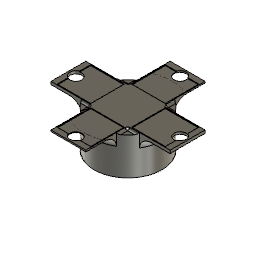
SpincoatG3P-8_rotor_4x_22x22coverslips_v1 (Autodesk Fusion 360 design; units mm, degrees)
Autodesk Fusion 360 part; units mm, degrees
sketch "Sketch1" plane through (0, 0, 0) normal (0, 0, 1) x (1, 0, 0)
  circle A0 centre (0, 0) radius 22.75
  dimension "d1" = 45.5
  constraint coincident A0.centre origin
  measures "d1" diameter of A0
extrude "Extrude1" add sketch "Sketch1" along normal blind 25
sketch "Sketch2" plane through (0, 0, 0) normal (0, 0, -1) x (1, 0, 0)
  circle A0 centre (0, 0) radius 22.75
  circle A1 centre (0, 0) radius 22.25
  dimension "d4" = 44.5
  constraint concentric A0 A1
  measures "d4" diameter of A1
extrude "Extrude2" cut sketch "Sketch2" against normal blind 10 contours A1
sketch "Sketch3" plane through (0, 0, 25) normal (0, 0, 1) x (-1, 0, 0)
  circle A0 centre (0, 0) radius 22.75
  line L0 (11.75, -27.5) -> (-11.75, -27.5)
  line L1 (-11.75, -27.5) -> (-11.75, 27.5)
  line L2 (-11.75, 27.5) -> (11.75, 27.5)
  line L3 (11.75, 27.5) -> (11.75, -27.5)
  line L4 (11.75, -27.5) -> (-11.75, 27.5) construction
  line L5 (-11.75, -27.5) -> (11.75, 27.5) construction
  dimension "d7" = 23.5
  dimension "d8" = 55
  constraint horizontal L0
  constraint perpendicular L0 L1
  constraint parallel L0 L2
  constraint parallel L1 L3
  constraint coincident L4 A0.centre
  constraint coincident L5 A0.centre
  constraint coincident A0.centre origin
  measures "d7" distance of L1.end L2.end
  measures "d8" distance of L0.end L1.end
sketch "Sketch6" plane through (0, 0, 25) normal (0, 0, 1) x (-1, 0, 0)
  circle A0 centre (0, 0) radius 22.75
  line L0 (-11.75, 40) -> (11.75, 40)
  line L1 (11.75, 40) -> (11.75, -40)
  line L2 (11.75, -40) -> (-11.75, -40)
  line L3 (-11.75, -40) -> (-11.75, 40)
  line L4 (-11.75, 40) -> (11.75, -40) construction
  line L5 (11.75, 40) -> (-11.75, -40) construction
  dimension "d17" = 23.5
  dimension "d18" = 80
  constraint horizontal L0
  constraint perpendicular L0 L1
  constraint parallel L0 L2
  constraint parallel L1 L3
  constraint coincident L4 A0.centre
  constraint coincident L5 A0.centre
  constraint coincident A0.centre origin
  measures "d17" distance of L1.end L2.end
  measures "d18" distance of L0.end L1.end
extrude "Extrude6" add sketch "Sketch6" along normal blind 1 contours A0 L1 L3 | A0 L0 L1 L3 | A0 L1 L2 L3
sketch "Sketch7" plane through (0, 0, 26) normal (0, 0, 1) x (-1, 0, 0)
  line L0 (-11.75, -40) -> (11.75, -40)
  line L1 (11.75, -40) -> (11.75, 40)
  line L2 (11.75, 40) -> (-11.75, 40)
  line L3 (-11.75, 40) -> (-11.75, -40)
  line L4 (-40, 11.75) -> (40, 11.75)
  line L5 (40, 11.75) -> (40, -11.75)
  line L6 (40, -11.75) -> (-40, -11.75)
  line L7 (-40, -11.75) -> (-40, 11.75)
  line L8 (-40, 11.75) -> (40, -11.75) construction
  line L9 (40, 11.75) -> (-40, -11.75) construction
  dimension "d21" = 80
  dimension "d22" = 23.5
  constraint horizontal L4
  constraint perpendicular L4 L5
  constraint parallel L4 L6
  constraint parallel L5 L7
  constraint coincident L8 origin
  constraint coincident L9 origin
  measures "d21" distance of L5.end L6.end
  measures "d22" distance of L4.end L5.end
extrude "Extrude7" add sketch "Sketch7" against normal blind 2 contours L3 L4 L6 L7 | L1 L3 L4 L6 | L1 L4 L5 L6
sketch "Sketch8" plane through (0, 0, 26) normal (0, 0, 1) x (-1, 0, 0)
  line L0 (11.75, 11.75) -> (11.75, 40)
  line L1 (11.75, 40) -> (-11.75, 40)
  line L2 (-11.75, 40) -> (-11.75, 11.75)
  line L3 (-11.75, 11.75) -> (-40, 11.75)
  line L4 (-40, 11.75) -> (-40, -11.75)
  line L5 (-40, -11.75) -> (-11.75, -11.75)
  line L6 (-11.75, -11.75) -> (-11.75, -40)
  line L7 (-11.75, -40) -> (11.75, -40)
  line L8 (11.75, -40) -> (11.75, -11.75)
  line L9 (11.75, -11.75) -> (40, -11.75)
  line L10 (40, -11.75) -> (40, 11.75)
  line L11 (40, 11.75) -> (11.75, 11.75)
  line L12 (-11.25, 36.25) -> (11.25, 36.25)
  line L13 (11.25, 36.25) -> (11.25, 13.75)
  line L14 (11.25, 13.75) -> (-11.25, 13.75)
  line L15 (-11.25, 13.75) -> (-11.25, 36.25)
  line L16 (-11.25, 36.25) -> (11.25, 13.75) construction
  line L17 (11.25, 36.25) -> (-11.25, 13.75) construction
  point P0 (0, 25)
  dimension "d25" = 22.5
  dimension "d26" = 22.5
  constraint horizontal L12
  constraint perpendicular L12 L13
  constraint parallel L12 L14
  constraint parallel L13 L15
  constraint coincident L16 P0
  constraint coincident L17 P0
  measures "d25" distance of L13.end L14.end
  measures "d26" distance of L12.end L13.end
extrude "Extrude8" cut sketch "Sketch8" against normal blind 0.5 contours L12 L13 L14 L15
sketch "Sketch9" plane through (0, 0, 26) normal (0, 0, 1) x (-1, 0, 0)
  line L0 (11.25, 36.25) -> (11.25, 13.75)
  line L1 (11.25, 13.75) -> (-11.25, 13.75)
  line L2 (-11.25, 13.75) -> (-11.25, 36.25)
  line L3 (-11.25, 36.25) -> (11.25, 36.25)
  line L4 (11.75, 11.75) -> (11.75, 40)
  line L5 (11.75, 40) -> (-11.75, 40)
  line L6 (-11.75, 40) -> (-11.75, 11.75)
  line L7 (-11.75, 11.75) -> (-40, 11.75)
  line L8 (-40, 11.75) -> (-40, -11.75)
  line L9 (-40, -11.75) -> (-11.75, -11.75)
  line L10 (-11.75, -11.75) -> (-11.75, -40)
  line L11 (-11.75, -40) -> (11.75, -40)
  line L12 (11.75, -40) -> (11.75, -11.75)
  line L13 (11.75, -11.75) -> (40, -11.75)
  line L14 (40, -11.75) -> (40, 11.75)
  line L15 (40, 11.75) -> (11.75, 11.75)
  line L16 (36.25, -11.25) -> (13.75, -11.25)
  line L17 (13.75, -11.25) -> (13.75, 11.25)
  line L18 (13.75, 11.25) -> (36.25, 11.25)
  line L19 (36.25, 11.25) -> (36.25, -11.25)
  line L20 (36.25, -11.25) -> (13.75, 11.25) construction
  line L21 (13.75, -11.25) -> (36.25, 11.25) construction
  point P0 (25, 0)
  dimension "d29" = 22.5
  dimension "d30" = 22.5
  constraint horizontal L16
  constraint perpendicular L16 L17
  constraint parallel L16 L18
  constraint parallel L17 L19
  constraint coincident L20 P0
  constraint coincident L21 P0
  measures "d29" distance of L17.end L18.end
  measures "d30" distance of L16.end L17.end
extrude "Extrude9" cut sketch "Sketch9" against normal blind 0.5 contours L16 L17 L18 L19
sketch "Sketch10" plane through (0, 0, 26) normal (0, 0, 1) x (-1, 0, 0)
  line L0 (13.75, -11.25) -> (13.75, 11.25)
  line L1 (13.75, 11.25) -> (36.25, 11.25)
  line L2 (36.25, 11.25) -> (36.25, -11.25)
  line L3 (36.25, -11.25) -> (13.75, -11.25)
  line L4 (11.25, 36.25) -> (11.25, 13.75)
  line L5 (11.25, 13.75) -> (-11.25, 13.75)
  line L6 (-11.25, 13.75) -> (-11.25, 36.25)
  line L7 (-11.25, 36.25) -> (11.25, 36.25)
  line L8 (11.75, 11.75) -> (11.75, 40)
  line L9 (11.75, 40) -> (-11.75, 40)
  line L10 (-11.75, 40) -> (-11.75, 11.75)
  line L11 (-11.75, 11.75) -> (-40, 11.75)
  line L12 (-40, 11.75) -> (-40, -11.75)
  line L13 (-40, -11.75) -> (-11.75, -11.75)
  line L14 (-11.75, -11.75) -> (-11.75, -40)
  line L15 (-11.75, -40) -> (11.75, -40)
  line L16 (11.75, -40) -> (11.75, -11.75)
  line L17 (11.75, -11.75) -> (40, -11.75)
  line L18 (40, -11.75) -> (40, 11.75)
  line L19 (40, 11.75) -> (11.75, 11.75)
  line L20 (-11.25, -36.25) -> (11.25, -36.25)
  line L21 (11.25, -36.25) -> (11.25, -13.75)
  line L22 (11.25, -13.75) -> (-11.25, -13.75)
  line L23 (-11.25, -13.75) -> (-11.25, -36.25)
  line L24 (-11.25, -36.25) -> (11.25, -13.75) construction
  line L25 (11.25, -36.25) -> (-11.25, -13.75) construction
  point P0 (0, -25)
  dimension "d33" = 22.5
  dimension "d34" = 22.5
  constraint horizontal L20
  constraint perpendicular L20 L21
  constraint parallel L20 L22
  constraint parallel L21 L23
  constraint coincident L24 P0
  constraint coincident L25 P0
  measures "d33" distance of L21.end L22.end
  measures "d34" distance of L20.end L21.end
extrude "Extrude10" cut sketch "Sketch10" against normal blind 0.5 contours L20 L21 L22 L23
sketch "Sketch11" plane through (0, 0, 26) normal (0, 0, 1) x (-1, 0, 0)
  line L0 (11.25, -36.25) -> (-11.25, -36.25)
  line L1 (-11.25, -36.25) -> (-11.25, -13.75)
  line L2 (-11.25, -13.75) -> (11.25, -13.75)
  line L3 (11.25, -13.75) -> (11.25, -36.25)
  line L4 (13.75, -11.25) -> (13.75, 11.25)
  line L5 (13.75, 11.25) -> (36.25, 11.25)
  line L6 (36.25, 11.25) -> (36.25, -11.25)
  line L7 (36.25, -11.25) -> (13.75, -11.25)
  line L8 (11.25, 36.25) -> (11.25, 13.75)
  line L9 (11.25, 13.75) -> (-11.25, 13.75)
  line L10 (-11.25, 13.75) -> (-11.25, 36.25)
  line L11 (-11.25, 36.25) -> (11.25, 36.25)
  line L12 (11.75, 11.75) -> (11.75, 40)
  line L13 (11.75, 40) -> (-11.75, 40)
  line L14 (-11.75, 40) -> (-11.75, 11.75)
  line L15 (-11.75, 11.75) -> (-40, 11.75)
  line L16 (-40, 11.75) -> (-40, -11.75)
  line L17 (-40, -11.75) -> (-11.75, -11.75)
  line L18 (-11.75, -11.75) -> (-11.75, -40)
  line L19 (-11.75, -40) -> (11.75, -40)
  line L20 (11.75, -40) -> (11.75, -11.75)
  line L21 (11.75, -11.75) -> (40, -11.75)
  line L22 (40, -11.75) -> (40, 11.75)
  line L23 (40, 11.75) -> (11.75, 11.75)
  line L24 (-36.25, 11.25) -> (-13.75, 11.25)
  line L25 (-13.75, 11.25) -> (-13.75, -11.25)
  line L26 (-13.75, -11.25) -> (-36.25, -11.25)
  line L27 (-36.25, -11.25) -> (-36.25, 11.25)
  line L28 (-36.25, 11.25) -> (-13.75, -11.25) construction
  line L29 (-13.75, 11.25) -> (-36.25, -11.25) construction
  point P0 (-25, 0)
  dimension "d37" = 22.5
  dimension "d38" = 22.5
  constraint horizontal L24
  constraint perpendicular L24 L25
  constraint parallel L24 L26
  constraint parallel L25 L27
  constraint coincident L28 P0
  constraint coincident L29 P0
  measures "d37" distance of L25.end L26.end
  measures "d38" distance of L24.end L25.end
extrude "Extrude11" cut sketch "Sketch11" against normal blind 0.5 contours L24 L25 L26 L27
sketch "Sketch12" plane through (0, 0, 24) normal (0, 0, -1) x (1, 0, 0)
  arc A0 (-19.4808, 11.75) -> (-19.4808, -11.75) centre (0, 0) ccw
  line L0 (-19.4808, 11.75) -> (-40, 11.75)
  line L1 (-40, 11.75) -> (-40, -11.75)
  line L2 (-40, -11.75) -> (-19.4808, -11.75)
  circle A1 centre (-35, 0) radius 4
  dimension "d41" = 8
  measures "d41" diameter of A1
extrude "Extrude12" cut sketch "Sketch12" against normal blind 10 contours A1
sketch "Sketch13" plane through (0, 0, 25) normal (0, 0, -1) x (1, 0, 0)
  arc A0 (11.75, 19.4808) -> (-11.75, 19.4808) centre (0, 0) ccw
  line L0 (11.75, 19.4808) -> (11.75, 40)
  line L1 (11.75, 40) -> (-11.75, 40)
  line L2 (-11.75, 40) -> (-11.75, 19.4808)
  circle A1 centre (0, 35) radius 4
  dimension "d44" = 8
  measures "d44" diameter of A1
extrude "Extrude13" cut sketch "Sketch13" against normal blind 10 contours A1
sketch "Sketch14" plane through (0, 0, 24) normal (0, 0, -1) x (1, 0, 0)
  arc A0 (19.4808, -11.75) -> (19.4808, 11.75) centre (0, 0) ccw
  line L0 (19.4808, -11.75) -> (40, -11.75)
  line L1 (40, -11.75) -> (40, 11.75)
  line L2 (40, 11.75) -> (19.4808, 11.75)
  circle A1 centre (35, 0) radius 4
  dimension "d47" = 8
  measures "d47" diameter of A1
extrude "Extrude14" cut sketch "Sketch14" against normal blind 10 contours A1
sketch "Sketch15" plane through (0, 0, 25) normal (0, 0, -1) x (1, 0, 0)
  arc A0 (-11.75, -19.4808) -> (11.75, -19.4808) centre (0, 0) ccw
  line L0 (-11.75, -19.4808) -> (-11.75, -40)
  line L1 (-11.75, -40) -> (11.75, -40)
  line L2 (11.75, -40) -> (11.75, -19.4808)
  circle A1 centre (0, -35) radius 4
  dimension "d50" = 8
  measures "d50" diameter of A1
extrude "Extrude15" cut sketch "Sketch15" against normal blind 10 contours A1
fillet "Fillet1" radius 7 1 edges at (-22.75, 0, 24)
fillet "Fillet2" radius 7 1 edges at (0, -22.75, 25)
fillet "Fillet3" radius 7 1 edges at (22.75, 0, 24)
fillet "Fillet4" radius 7 1 edges at (0, 22.75, 25)
fillet "Fillet5" radius 2 1 edges at (-15.6154, -11.75, 25)
fillet "Fillet6" radius 2 2 edges at (-11.75, -16.4814, 25) (-11.75, -12.4821, 25.2679)
fillet "Fillet7" radius 2 1 edges at (11.75, -15.6154, 25)
fillet "Fillet8" radius 2 2 edges at (16.4814, -11.75, 25) (12.4821, -11.75, 25.2679)
fillet "Fillet9" radius 2 1 edges at (15.6154, 11.75, 25)
fillet "Fillet10" radius 2 2 edges at (11.75, 16.4814, 25) (11.75, 12.4821, 25.2679)
fillet "Fillet11" radius 2 1 edges at (-11.75, 15.6154, 25)
fillet "Fillet12" radius 2 2 edges at (-16.4814, 11.75, 25) (-12.4821, 11.75, 25.2679)
extrude "Extrude3" [suppressed]
sketch "Sketch4" plane through (0, 0, 25) normal (0, 0, 1) x (-1, 0, 0)
  line L0 (-11.75, -19.4808) -> (-11.75, 19.4808)
  arc A0 (-11.75, 19.4808) -> (-11.75, -19.4808) centre (0, 0) ccw
  line L1 (27.5, -11.75) -> (-27.5, -11.75)
  line L2 (-27.5, -11.75) -> (-27.5, 11.75)
  line L3 (-27.5, 11.75) -> (27.5, 11.75)
  line L4 (27.5, 11.75) -> (27.5, -11.75)
  line L5 (27.5, -11.75) -> (-27.5, 11.75) construction
  line L6 (-27.5, -11.75) -> (27.5, 11.75) construction
  dimension "d11" = 55
  dimension "d12" = 23.5
  constraint horizontal L1
  constraint perpendicular L1 L2
  constraint parallel L1 L3
  constraint parallel L2 L4
  constraint coincident L5 A0.centre
  constraint coincident L6 A0.centre
  constraint coincident A0.centre origin
  measures "d11" distance of L2.end L3.end
  measures "d12" distance of L1.end L2.end
extrude "Extrude4" [suppressed]
extrude "Extrude5" [suppressed]
sketch "Sketch5" plane through (0, 0, 25.5) normal (0, 0, 1) x (-1, 0, 0)
  line L0 (-11.75, -11.75) -> (-11.75, -27.5)
  line L1 (-11.75, -27.5) -> (11.75, -27.5)
  line L2 (11.75, -27.5) -> (11.75, -11.75)
  line L3 (11.75, -11.75) -> (27.5, -11.75)
  line L4 (27.5, -11.75) -> (27.5, 11.75)
  line L5 (27.5, 11.75) -> (11.75, 11.75)
  line L6 (11.75, 11.75) -> (11.75, 27.5)
  line L7 (11.75, 27.5) -> (-11.75, 27.5)
  line L8 (-11.75, 27.5) -> (-11.75, 11.75)
  line L9 (-11.75, 11.75) -> (-27.5, 11.75)
  line L10 (-27.5, 11.75) -> (-27.5, -11.75)
  line L11 (-27.5, -11.75) -> (-11.75, -11.75)
